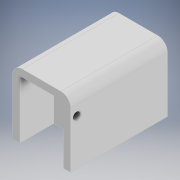
# Autodesk Inventor part: Case_Side
Saved by Autodesk Inventor 2020 (Build 240168000, 168)
## iProperties
Created: 2019-11-07
Part Number: Case_Side
Material: 일반
Document SubType Name: Modeling
Designer: Knowblesse
Density: 1 g/cm^3
Appearance: 기본값
Author: Knowblesse
## iProperties of the stored document _3D 인쇄.ipt
Created: 2019-11-07
Part Number: _3D 인쇄
Material: 일반
Document SubType Name: Modeling
Designer: Knowblesse
Density: 1 g/cm^3
Appearance: 기본값
Author: Knowblesse
Autodesk Inventor part; units mm, degrees
ref_plane "YZ Plane" through (0, 0, 0) normal (1, 0, 0) x (0, 1, 0)
ref_plane "XZ Plane" through (0, 0, 0) normal (0, 1, 0) x (-1, 0, 0)
ref_plane "XY Plane" through (0, 0, 0) normal (0, 0, 1) x (1, 0, 0)
sketch "스케치1" plane through (0, 0, 0) normal (0, 0, 1) x (1, 0, 0)
  line L0 (0, 0) -> (9, 0)
  line L1 (9, 0) -> (9, 10.5)
  line L2 (9, 10.5) -> (0, 10.5)
  line L3 (0, 10.5) -> (0, 0)
  line L4 (-1.5, 12) -> (10.5, 12)
  line L5 (10.5, 12) -> (10.5, -1.5)
  line L6 (10.5, -1.5) -> (-1.5, -1.5)
  line L7 (-1.5, -1.5) -> (-1.5, 12)
  line L8 (0, 0) -> (0, -1.5)
  line L9 (9, 0) -> (9, -1.5)
  line L10 (0, 0) -> (-1.5, 0)
  line L11 (9, 0) -> (10.5, 0)
  dimension "d0" = 9
  dimension "d1" = 10.5
  dimension "d2" = 1.5
  constraints: 24 end point, 6 point on line, 4 parallel, 4 perpendicular, 1 horizontal, 3 other
  measures "d0" distance of L2.end L1.end
  measures "d1" distance of L1.end L0.end
  measures "d2" distance between parallel lines of L2 L4
extrude "돌출1" add sketch "스케치1" along normal blind 20 contours L10 L7 L4 L5 L11 L1 L2 L3 | L8 L6 L7 L10 | L11 L5 L6 L9
sketch "스케치2" plane through (-1.5, -1.5, 0) normal (0, -1, 0) x (1, 0, 0)
  line L0 (0, 0) -> (1.5, 0) projected
  line L1 (1.5, 0) -> (1.5, 20) projected
  line L2 (0, 20) -> (1.5, 20) projected
  line L3 (0, 0) -> (0, 20) projected
  line L4 (1.5, 5) -> (0, 5)
  line L5 (0, 5) -> (0, 6)
  line L6 (0, 6) -> (1.5, 6)
  line L7 (1.5, 6) -> (1.5, 5)
  point P0 (1.5, 0)
  point P1 (1.5, 6)
  point P2 (0, 5)
  dimension "d5" = 1
  dimension "d6" = 5
  constraints: 8 end point, 2 parallel, 2 point on line, 1 horizontal, 1 perpendicular
  measures "d5" distance of L4.end L5.end
  measures "d6" distance between parallel lines of L4 L0
extrude "돌출2" cut sketch "스케치2" against normal blind 8 contours L3 L6 L1 L4
fillet "모깎기1" radius 2 2 edges at (-1.5, 12, 10) (10.5, 12, 10)
sketch "스케치5" plane through (0, 10.5, 0) normal (0, -1, 0) x (1, 0, 0)
  line L0 (0, 0) -> (9, 0) projected
  line L1 (9, 0) -> (9, 20) projected
  line L2 (0, 20) -> (9, 20) projected
  line L3 (0, 0) -> (0, 20) projected
  line L4 (9, 17.5) -> (7, 17.5)
  line L5 (7, 17.5) -> (7, 20)
  line L6 (8.5, 20) -> (0.5, 20) projected
  point P0 (0, 0)
  dimension "d21" = 2.5
  dimension "d22" = 2
  constraints: 4 end point, 2 point on line, 1 horizontal, 1 perpendicular
  measures "d21" distance between parallel lines of L2 L4
  measures "d22" distance between parallel lines of L5 L1
extrude "돌출5" add sketch "스케치5" along normal blind 5 contours L4 L5 L2 L1
sketch "스케치6" plane through (7, 10.5, 17.5) normal (-1, 0, 0) x (0, 0, 1)
  line L0 (2.5, -5) -> (0, -5) projected
  line L1 (-17.5, 0) -> (0, 0) projected
  point P0 (-17.5, -10.5)
  point P1 (1.25, -2.5)
  point P2 (1.25, -5)
  dimension "d25" = 2.5
  constraints: 1 midpoint, 1 vertical alignment
  measures "d25" distance from line of L1 point (1.25, -2.5)
hole "구멍1" at (7, 8, 18.75) direction (1, 0, 0) diameter 1.5 end through all
